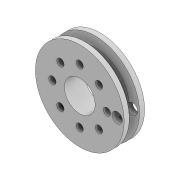
# Autodesk Inventor part: Motor_pulley
Saved by Autodesk Inventor 2022 (Build 260153000, 153)
## iProperties
Created: 2022-07-09
Part Number: Motor_pulley
Material: Generic
Document SubType Name: Modeling
Designer: dell
Density: 1 g/cm^3
Appearance: Default
Author: dell
Autodesk Inventor part; units mm, degrees
ref_plane "YZ Plane" through (0, 0, 0) normal (1, 0, 0) x (0, 1, 0)
ref_plane "XZ Plane" through (0, 0, 0) normal (0, 1, 0) x (-1, 0, 0)
ref_plane "XY Plane" through (0, 0, 0) normal (0, 0, 1) x (1, 0, 0)
sketch "Sketch1" plane through (0, 0, 0) normal (1, 0, 0) x (0, 1, 0)
  line L0 (0, 3) -> (13, 3)
  line L1 (13, 3) -> (13, -3)
  line L2 (13, -3) -> (0, -3)
  line L3 (0, -3) -> (0, 3)
  line L4 (0, -4.2) -> (0, 4.2) projected
  line L5 (13, 1.5) -> (13, -1.5)
  line L6 (13, -1.5) -> (10, -1.5)
  line L7 (10, -1.5) -> (10, 1.5)
  line L8 (10, 1.5) -> (13, 1.5)
  point P0 (0, 0)
  dimension "d0" = 6
  dimension "d1" = 3
  dimension "d2" = 13
  dimension "d4" = 1.5
  dimension "d5" = 1.5
  dimension "d19" = 3
  constraints: 16 end point, 4 parallel, 2 perpendicular, 2 point on line, 1 horizontal, 1 midpoint, 1 vertical
  measures "d0" distance of L2.end L0.start
  measures "d1" distance from line of point (0, 0) L0
  measures "d2" distance between parallel lines of L1 L3
  measures "d4" distance from line of L0 L5.start
  measures "d5" distance of L1.end L5.end
  measures "d19" distance of L5.end L6.end
revolve "Revolution1" add sketch "Sketch1" angle 360 about axis through (0, 0, -10) along (0, 0, 1) contours L0 L1 L8 L7 L6 L2 L3
sketch "Sketch2" plane through (0, 0, -3) normal (0, 0, -1) x (-1, 0, 0)
  circle A0 centre (0, 8) radius 1.05
  circle A1 centre (0, 0) radius 4.5
  dimension "d7" = 2.1
  dimension "d8" = 8
  dimension "d9" = 9
  constraints: 2 centre point, 1 coincident
  measures "d7" diameter of A0
  measures "d8" distance of point (0, 0) A0.centre
  measures "d9" diameter of A1
extrude "Extrusion1" cut sketch "Sketch2" against normal blind 100
pattern_circular "Circular Pattern1" count 8 over 360 about axis through (0, 0, -10) along (0, 0, 1) of "Extrusion1"
sketch "Sketch3" plane through (0, 0, -3) normal (0, 0, -1) x (-1, 0, 0)
  circle A0 centre (-11, 0) radius 1.5
  point P0 (0, 0)
  dimension "d15" = 3
  dimension "d16" = 11
  constraints: 1 centre point
  measures "d15" diameter of A0
  measures "d16" distance of point (0, 0) A0.centre
extrude "Extrusion2" cut sketch "Sketch3" against normal blind 100
body "Solid1"
